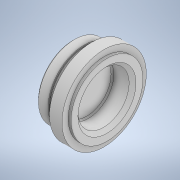
# Autodesk Inventor part: Крышка_пром
Saved by Autodesk Inventor 2021 (Build 250183000, 183)
## iProperties
Created: 2023-03-17
Part Number: Крышка_пром
Material: Типовые
Document SubType Name: Modeling
Designer: gdevc
Density: 1 g/cm^3
Appearance: По умолчанию
Mass: 40.1447 g
Surface Area: 108.148 cm^2
Volume: 40.1447 cm^3
Author: gdevc
Autodesk Inventor part; units mm, degrees
ref_plane "YZ Plane" through (0, 0, 0) normal (1, 0, 0) x (0, 1, 0)
ref_plane "XZ Plane" through (0, 0, 0) normal (0, 1, 0) x (-1, 0, 0)
ref_plane "XY Plane" through (0, 0, 0) normal (0, 0, 1) x (1, 0, 0)
sketch "Эскиз1" plane through (0, 0, 0) normal (0, 0, 1) x (1, 0, 0)
  line L0 (0, 0) -> (0, 26)
  line L1 (0, 26) -> (8, 26)
  line L2 (8, 26) -> (8.5, 25.5)
  line L3 (8.5, 25.5) -> (13.5, 25.5)
  line L4 (13.5, 25.5) -> (13.5, 30.5)
  line L5 (13.5, 30.5) -> (22.5, 30.5)
  line L6 (22.5, 30.5) -> (22.5, 26)
  line L7 (22.5, 18.5) -> (10, 18.5)
  line L8 (10, 18.5) -> (10, 0)
  line L9 (10, 0) -> (0, 0)
  line L10 (22.5, 26) -> (24.55, 26)
  line L11 (24.55, 26) -> (24.55, 18.5)
  line L12 (24.55, 18.5) -> (22.5, 18.5)
  dimension "d0" = 52
  dimension "d1" = 0.5
  dimension "d2" = 45
  dimension "d3" = 5
  dimension "d4" = 8
  dimension "d5" = 12
  dimension "d6" = 10
  dimension "d7" = 9
  dimension "d8" = 4.5
  dimension "d19" = 22.5
  dimension "d23" = 2.05
  constraints: 26 end point, 9 perpendicular, 1 horizontal, 1 parallel, 1 point on line, 1 vertical
  measures "d0" diameter of L1 L9
  measures "d1" distance between parallel lines of L1 L3
  measures "d2" angle of L3 L2
  measures "d3" distance of L2.end L3.end
  measures "d4" distance of L0.end L1.end
  measures "d5" distance between parallel lines of L7 L5
  measures "d6" distance between parallel lines of L0 L8
  measures "d7" distance of L4.end L5.end
  measures "d8" distance between parallel lines of L1 L5
  measures "d19" distance between parallel lines of L6 L0
  measures "d23" distance of L6.end L10.end
revolve "Вращение1" add sketch "Эскиз1" angle 360 about axis through (10, 0, 0) along (-1, 0, 0)
fillet "Сопряжение1" radius 0.5 1 edges at (8.5, -25.5, 0)
fillet "Сопряжение2" radius 1.6 1 edges at (13.5, -25.5, 0)
chamfer "Фаска1" distance 1 angle 45 1 edges at (0, -26, 0)
fillet "Сопряжение3" radius 1 1 edges at (10, -18.5, 0)
chamfer "Фаска4" distance 2.5 angle 45 1 edges at (24.55, -18.5, 0)
equation "\"d5\" = 1.5 * d4"
equation "\"d8\" = 0.5 * d7"
